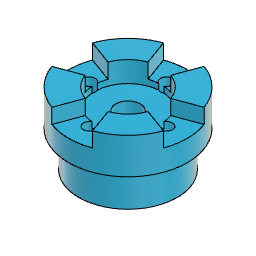
Assemblage_croix_de_malte_KOSMOS3-0 (Autodesk Fusion 360 archive; units mm, degrees)
design "extrémité croix de malte v7"
Autodesk Fusion 360 part; units mm, degrees
sketch "Esquisse1" plane through (0, 0, 0) normal (0, 0, 1) x (1, 0, 0)
  circle A0 centre (0, 0) radius 16.55
  circle A1 centre (0, 0) radius 4.1
  circle A2 centre (-13, 0) radius 2
  circle A3 centre (0, -13) radius 2
  circle A4 centre (13, 0) radius 2
  circle A5 centre (0, 13) radius 2
  dimension "d1" = 33.1
  dimension "d2" = 8.2
  dimension "d3" = 4
  dimension "d4" = 13
  dimension "d6" = 360
  constraint coincident A0.centre A1.centre
  constraint concentric A0 A1
  measures "d1" diameter of A0
  measures "d2" diameter of A1
  measures "d3" diameter of A2
  measures "d4" distance of A0.centre A2.centre
extrude "Extrusion1" add sketch "Esquisse1" along normal blind 19
sketch "Esquisse2" plane through (0, 0, 0) normal (0, 0, -1) x (1, 0, 0)
  circle A0 centre (13, 0) radius 2
  circle A1 centre (-13, 0) radius 2
  circle A2 centre (0, 0) radius 4.1
  circle A3 centre (0, 13) radius 2
  circle A4 centre (0, -13) radius 2
  circle A5 centre (0, 0) radius 16.55
hole "Perçage1" at (0, -13, 0) direction (0, 0, 1) diameter 6 depth 4 tip angle 180
hole "Perçage2" at (-13, 0, 0) direction (0, 0, 1) diameter 6 depth 4 tip angle 180
hole "Perçage3" at (13, 0, 0) direction (0, 0, 1) diameter 6 depth 4 tip angle 180
hole "Perçage4" at (0, 13, 0) direction (0, 0, 1) diameter 6 depth 4 tip angle 180
hole "Perçage5" at (0, 0, 19) direction (0, 0, -1) diameter 22.5 depth 2 tip angle 180
sketch "Esquisse3" plane through (0, 0, 19) normal (0, 0, 1) x (-1, 0, 0)
  circle A0 centre (0, 0) radius 16.55
  arc A1 (11.2139, 0.9) -> (0.9, 11.2139) centre (0, 0) ccw
  arc A2 (11.2139, -0.9) -> (11.2139, 0.9) centre (13, 0) ccw
  arc A3 (0.9, -11.2139) -> (11.2139, -0.9) centre (0, 0) ccw
  arc A4 (-0.9, -11.2139) -> (0.9, -11.2139) centre (0, -13) ccw
  arc A5 (-11.2139, -0.9) -> (-0.9, -11.2139) centre (0, 0) ccw
  arc A6 (-11.2139, 0.9) -> (-11.2139, -0.9) centre (-13, 0) ccw
  arc A7 (-0.9, 11.2139) -> (-11.2139, 0.9) centre (0, 0) ccw
  arc A8 (0.9, 11.2139) -> (-0.9, 11.2139) centre (0, 13) ccw
  circle A9 centre (0, 0) radius 20
  dimension "d24" = 40
  constraint concentric A0 A9
  measures "d24" diameter of A9
extrude "Extrusion2" add sketch "Esquisse3" against normal blind 7.1 contours A9
sketch "Esquisse4" plane through (0, 0, 19) normal (0, 0, 1) x (-1, 0, 0)
  circle A0 centre (0, 0) radius 20
  arc A1 (11.2139, 0.9) -> (0.9, 11.2139) centre (0, 0) ccw
  arc A2 (11.2139, -0.9) -> (11.2139, 0.9) centre (13, 0) ccw
  arc A3 (0.9, -11.2139) -> (11.2139, -0.9) centre (0, 0) ccw
  arc A4 (-0.9, -11.2139) -> (0.9, -11.2139) centre (0, -13) ccw
  arc A5 (-11.2139, -0.9) -> (-0.9, -11.2139) centre (0, 0) ccw
  arc A6 (-11.2139, 0.9) -> (-11.2139, -0.9) centre (-13, 0) ccw
  arc A7 (-0.9, 11.2139) -> (-11.2139, 0.9) centre (0, 0) ccw
  arc A8 (0.9, 11.2139) -> (-0.9, 11.2139) centre (0, 13) ccw
  line L0 (0, 0) -> (14.1421, -14.1421) construction
  line L1 (0, 0) -> (20, 0) construction
  line L2 (0, 0) -> (18.7939, -6.8404) construction
  line L3 (0, 0) -> (6.8404, -18.7939) construction
  line L4 (0, 0) -> (20, 0) construction
  line L5 (18.7939, -6.8404) -> (10.5715, -3.8477)
  line L6 (6.8404, -18.7939) -> (3.8477, -10.5715)
  arc A9 (3.8477, -10.5715) -> (10.5715, -3.8477) centre (0, 0) ccw
  arc A10 (6.8404, -18.7939) -> (18.7939, -6.8404) centre (0, 0) ccw
  arc A11 (10.5715, 3.8477) -> (3.8477, 10.5715) centre (0, 0) ccw
  line L7 (6.8404, 18.7939) -> (3.8477, 10.5715)
  arc A12 (18.7939, 6.8404) -> (6.8404, 18.7939) centre (0, 0) ccw
  line L8 (18.7939, 6.8404) -> (10.5715, 3.8477)
  arc A13 (-3.8477, 10.5715) -> (-10.5715, 3.8477) centre (0, 0) ccw
  line L9 (-18.7939, 6.8404) -> (-10.5715, 3.8477)
  arc A14 (-6.8404, 18.7939) -> (-18.7939, 6.8404) centre (0, 0) ccw
  line L10 (-6.8404, 18.7939) -> (-3.8477, 10.5715)
  arc A15 (-10.5715, -3.8477) -> (-3.8477, -10.5715) centre (0, 0) ccw
  line L11 (-6.8404, -18.7939) -> (-3.8477, -10.5715)
  arc A16 (-18.7939, -6.8404) -> (-6.8404, -18.7939) centre (0, 0) ccw
  line L12 (-18.7939, -6.8404) -> (-10.5715, -3.8477)
  dimension "d27" = 45
  dimension "d28" = 25
  dimension "d29" = 70
  dimension "d31" = 360
  constraint horizontal L1
  constraint coincident A0.centre A1.centre
  constraint coincident A0 L2.end
  constraint horizontal L4
  constraint coincident A3 L5.end
  constraint coincident L2 L5.end
  constraint coincident A3 L6.end
  constraint coincident L3 L6.end
  measures "d27" angle of L0 L1
  measures "d28" angle of L0 L2
  measures "d29" angle of L3 L4
extrude "Extrusion3" add sketch "Esquisse4" along normal blind 5 contours A0 A1 A11 L7 A12 L8 | A0 A3 L5 L6 A9 A10 | A0 A7 A13 L9 A14 L10 | A0 A5 A15 L11 A16 L12
